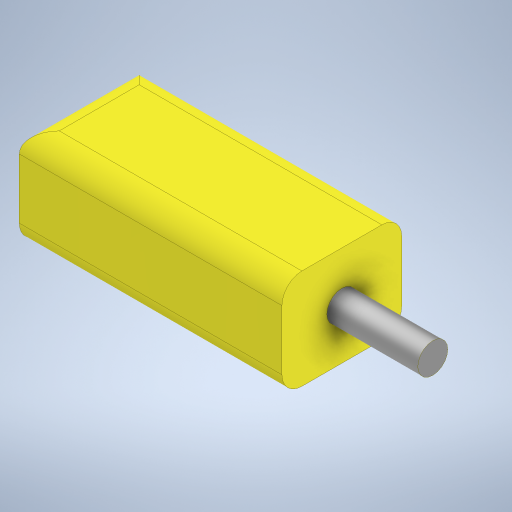
# Autodesk Inventor part: motor
Saved by Autodesk Inventor 2024 (Build 280153000, 153)
## iProperties
Created: 2023-10-20
Part Number: motor
Material: Aluminum 6061
Document SubType Name: Modeling
Designer: kdcao
Density: 2.7 g/cm^3
Appearance: Canary
Author: kdcao
Autodesk Inventor part; units mm, degrees
ref_plane "YZ Plane" through (0, 0, 0) normal (1, 0, 0) x (0, 1, 0)
ref_plane "XZ Plane" through (0, 0, 0) normal (0, 1, 0) x (-1, 0, 0)
ref_plane "XY Plane" through (0, 0, 0) normal (0, 0, 1) x (1, 0, 0)
sketch "Sketch1" plane through (0, 0, 0) normal (1, 0, 0) x (0, 1, 0)
  line L0 (-5, 6) -> (5, 6)
  line L1 (5, 6) -> (5, -6)
  line L2 (5, -6) -> (-5, -6)
  line L3 (-5, -6) -> (-5, 6)
  line L4 (-5, 6) -> (5, -6) construction
  line L5 (5, 6) -> (-5, -6) construction
  point P0 (0, 0)
  dimension "d0" = 10
  dimension "d1" = 12
  constraints: 12 end point, 2 midpoint, 2 parallel, 1 horizontal, 1 perpendicular
  measures "d0" distance of L0.start L0.end
  measures "d1" distance of L0.end L1.end
extrude "Extrusion1" add sketch "Sketch1" along normal blind 26.29
sketch "Sketch2" plane through (26.29, 0, 0) normal (1, 0, 0) x (0, 0, -1)
  circle A0 centre (0, 0) radius 1.5
  dimension "d4" = 3
  constraints: 1 centre point, 1 coincident
  measures "d4" diameter of A0
fillet "Fillet1" radius 2 5 edges at (13.145, 5, 6) (13.145, 5, -6) (13.145, -5, 6) (13.145, -5, -6) (0, 5, 0)
extrude "Extrusion2" add sketch "Sketch2" along normal blind 9.1
body "Solid1"
